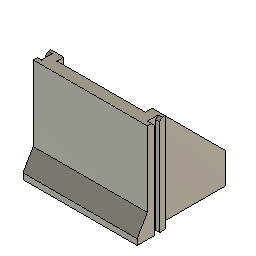
Caliper Battery Door (Autodesk Fusion 360 design; units mm, degrees)
Autodesk Fusion 360 part; units mm, degrees
sketch "Sketch1" plane through (0, 0, 0) normal (0, 0, 1) x (1, 0, 0)
  line L0 (0, 0) -> (-0.9251, 0)
  line L1 (-0.6, -0.8) -> (0, -0.8)
  line L2 (0, -0.8) -> (0, 0)
  line L3 (-0.6, -0.8) -> (-0.6, -1.6)
  line L4 (-0.6, -1.6) -> (0, -1.6)
  line L5 (0, -1.6) -> (0, -2.6)
  line L6 (-8.4, -2.6) -> (-8.4, -0.0952)
  line L7 (-16.8, -1.6) -> (-16.8, -2.6)
  line L8 (-16.2, -1.6) -> (-16.8, -1.6)
  line L9 (-16.2, -0.8) -> (-16.2, -1.6)
  line L10 (-16.2, -0.8) -> (-16.8, -0.8)
  line L11 (-16.8, -0.8) -> (-16.8, 0)
  line L12 (-16.8, -2.6) -> (-8.4, -2.6)
  line L13 (-16.8, 0) -> (0, 0)
  line L14 (0, -2.6) -> (-16.8, -2.6)
  dimension "d1" = 1
  dimension "d2" = 0.8
  dimension "d3" = 0.8
  dimension "d4" = 0.6
  dimension "d6" = 16.8
  constraint horizontal L0
  constraint horizontal L1
  constraint vertical L2
  constraint coincident L0.start L2.end
  constraint perpendicular L1 L3
  constraint perpendicular L2 L4
  constraint perpendicular L4 L5
  constraint perpendicular L0 L6
  constraint symmetric L0.start L6 L11.end
  constraint symmetric L1.start L6 L9.start
  constraint symmetric L1.end L6 L10.end
  constraint symmetric L3.end L6 L8.start
  constraint symmetric L4.end L6 L7.start
  constraint symmetric L5.end L6 L7.end
  constraint symmetric L12.end L6 L6.start
  constraint midpoint L6.start L14
  constraint collinear L2 L5
  measures "d1" distance of L4.end L5.end
  measures "d2" distance of L0.start L1.end
  measures "d3" distance of L1.start L3.end
  measures "d4" distance of L3.end L4.end
  measures "d6" distance of L5.end L7.end
extrude "Extrude1" add sketch "Sketch1" along normal blind 14.5
sketch "Sketch2" plane through (0, 0, 0) normal (1, 0, 0) x (0, 1, 0)
  line L0 (-2.6, 0) -> (-1.6, 0)
  line L1 (-1.6, 0) -> (-1.6, 14.5)
  line L2 (-1.6, 14.5) -> (-2.6, 14.5)
  line L3 (-2.6, 14.5) -> (-2.6, 0)
  line L4 (-2.6, 0) -> (-2.6, 14.5)
  line L5 (-1.6, 0) -> (-2.6, 0)
  line L6 (-2.6, 0) -> (-4.6, 0)
  line L7 (-4.6, 0) -> (-2.6, 3.4641)
  line L8 (-4.1, 0) -> (-4.1, 0.866)
  point P0 (-2.6, 0)
  dimension "d9" = 60
  dimension "d10" = 2
  dimension "d17" = 1.5
  constraint coincident P0 L0.start
  constraint perpendicular L4 L6
  constraint coincident L3 L7.end
  constraint coincident L6 L8.start
  constraint coincident L7 L8.end
  constraint perpendicular L6 L8
  measures "d9" angle of L6 L7
  measures "d10" distance of P0 L6.end
  measures "d17" distance of L8.start P0
extrude "Extrude2" add sketch "Sketch2" against normal blind 16.8 contours L3 L4 L6 L7 L8
sketch "Sketch3" plane through (0, 0, 0) normal (0, 1, 0) x (-1, 0, 0)
  line L0 (0, 0) -> (16.8, 0)
  line L1 (16.8, 0) -> (16.8, 14.5)
  line L2 (16.8, 14.5) -> (0, 14.5)
  line L3 (0, 14.5) -> (0, 0)
  line L4 (0, 14.5) -> (16.8, 14.5)
  line L5 (8.4, 14.5) -> (8.4, 8) construction
  line L6 (1.9, 14.5) -> (1.9, 8)
  line L7 (14.9, 14.5) -> (14.9, 8)
  arc A0 (1.9, 8) -> (14.9, 8) centre (8.4, 8) ccw
  dimension "d13" = 6.5
  dimension "d14" = 13
  constraint midpoint L4 L5.start
  constraint perpendicular L4 L5
  constraint coincident L5.end A0.centre
  constraint coincident L2 L6.start
  constraint tangent L6 A0
  constraint vertical L6
  constraint symmetric L5 L6.start L7.start
  constraint symmetric L5 L6.end L7.end
  measures "d13" distance of L5.start L5.end
  measures "d14" diameter of A0
extrude "Extrude3" cut sketch "Sketch3" against normal blind 1 contours L2 L4 L6 L7 A0
chamfer "Chamfer1" distance 0.4 angle 45 4 edges at (-16.5, -0.8, 14.5) (-16.5, -1.6, 14.5) (-0.3, -0.8, 14.5) (-0.3, -1.6, 14.5)
sketch "Sketch4" plane through (0, 0, 0) normal (0, 1, 0) x (-1, 0, 0)
  line L0 (1.9, 8) -> (1.9, 14.5)
  line L1 (1.9, 14.5) -> (0, 14.5)
  line L2 (0, 14.5) -> (0, 0)
  line L3 (0, 0) -> (16.8, 0)
  line L4 (16.8, 0) -> (16.8, 14.5)
  line L5 (16.8, 14.5) -> (14.9, 14.5)
  line L6 (14.9, 14.5) -> (14.9, 8)
  arc A0 (1.9, 8) -> (14.9, 8) centre (8.4, 8) ccw
  line L7 (1.9, 14.5) -> (1.9, 0)
  line L8 (1.1, 0) -> (1.1, 14.5)
  dimension "d19" = 0.8
  constraint coincident L0.end L1.start
  constraint coincident L3 L7.end
  constraint perpendicular L3 L7
  constraint coincident L3 L8.start
  constraint coincident L1 L8.end
  constraint parallel L7 L8
  measures "d19" distance of L0.end L8.end
extrude "Extrude4" add sketch "Sketch4" along normal blind 10 contours L0 L1 L3 L7 L8
chamfer "Chamfer2" distance 10 angle 45 1 edges at (-1.5, 10, 14.5)
named bodies: "Caliper Battery door"
